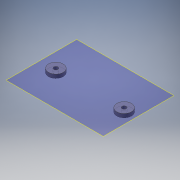
# Autodesk Inventor part: ChassisPrototypeA3
Saved by Autodesk Inventor 2017 (Build 210142000, 142)
## iProperties
Created: 2018-04-24
Part Number: ChassisPrototypeA3
Material: Generic
Document SubType Name: Modeling
Designer: MtgSaber
Mass: 3.50044 g
Surface Area: 26.3822 cm^2
Volume: 3.50044 cm^3
Density: 1 g/cm^3
Appearance: Default
Author: MtgSaber
Autodesk Inventor part; units mm, degrees
ref_plane "YZ Plane" through (0, 0, 0) normal (1, 0, 0) x (0, 1, 0)
ref_plane "Work Plane1" through (-38.4302, 0, 40.64) normal (0, -1, 0) x (-1, 0, 0)
sketch "Sketch1" plane through (-38.4302, 0, 40.64) normal (0, -1, 0) x (-1, 0, 0)
  circle A0 centre (29.6799, 0) radius 1.8288 construction
  circle A1 centre (-29.6799, 0) radius 1.8288 construction
  line L0 (-34.4805, -7.5946) -> (34.4805, -7.5946) construction
  line L1 (34.4805, -7.5946) -> (34.4805, -19.2786) construction
  line L2 (34.4805, -19.2786) -> (-34.4805, -19.2786) construction
  line L3 (-34.4805, -19.2786) -> (-34.4805, -7.5946) construction
  line L4 (34.4805, 7.5946) -> (-34.4805, 7.5946) construction
  line L5 (-34.4805, 7.5946) -> (-34.4805, 19.2786) construction
  line L6 (-34.4805, 19.2786) -> (34.4805, 19.2786) construction
  line L7 (34.4805, 19.2786) -> (34.4805, 7.5946) construction
  line L8 (-38.4302, 27.94) -> (38.4302, 27.94) construction
  line L9 (-38.4302, -27.94) -> (-38.4302, 27.94) construction
  line L10 (38.4302, -27.94) -> (-38.4302, -27.94) construction
  line L11 (38.4302, 27.94) -> (38.4302, -27.94) construction
  circle A2 centre (-29.6799, 0) radius 1.8288
  circle A3 centre (29.6799, 0) radius 1.8288
  circle A4 centre (29.6799, 0) radius 6.35
  circle A5 centre (-29.6799, 0) radius 6.35
  point P0 (-38.4302, 40.64)
  dimension "d0" = 12.7
  dimension "d1" = 12.7
  constraints: 4 centre point, 4 coincident, 2 concentric
  measures "d0" diameter of A4
  measures "d1" diameter of A5
extrude "Extrusion1" add sketch "Sketch1" along normal blind 3.175
ref_plane "Work Plane2" through (-76.8604, 0, 40.64) normal (0, 0, 1) x (1, 0, 0)
sketch "Sketch2" plane through (-76.8604, 0, 40.64) normal (0, 0, 1) x (1, 0, 0)
  line L0 (10.5791, -3.175) -> (6.9215, -3.175) construction
  line L1 (6.9215, 0) -> (10.5791, 0) construction
  line L2 (69.9389, -3.175) -> (66.2813, -3.175) construction
  line L3 (66.2813, 0) -> (69.9389, 0) construction
  line L4 (6.9215, 0) -> (10.5791, 0) construction
  line L5 (8.7503, 0) -> (68.1101, 0) construction
  line L6 (-4.3871, -3.175) -> (85.3512, -3.175) construction
  circle A0 centre (38.4302, -9.525) radius 2.0574
  circle A1 centre (38.4302, -9.525) radius 6.35 construction
  line L7 (38.4302, 0) -> (38.4302, -31.2723) construction
  circle A2 centre (51.1302, -9.525) radius 2.0574
  arc A3 (51.1302, -15.875) -> (57.4802, -9.525) centre (51.1302, -9.525) ccw
  circle A4 centre (25.7302, -9.525) radius 2.0574
  arc A5 (19.3802, -9.525) -> (25.7302, -15.875) centre (25.7302, -9.525) ccw
  line L8 (25.7302, -15.875) -> (51.1302, -15.875)
  line L9 (19.3802, -3.175) -> (57.4802, -3.175)
  line L10 (19.3802, -9.525) -> (19.3802, -3.175)
  line L11 (57.4802, -9.525) -> (57.4802, -3.175)
  point P0 (76.8604, 0)
  point P1 (25.7302, -3.175)
  point P2 (51.1302, -3.175)
  dimension "d4" = 3.175
  dimension "d5" = 4.1148
  dimension "d6" = 12.7
  dimension "d7" = 4.1148
  dimension "d8" = 12.7
  constraints: 14 end point, 7 point on line, 6 centre point, 6 tangent, 4 point on circle, 3 coincident, 3 midpoint, 2 horizontal, 2 perpendicular, 2 symmetric about line, 1 parallel, 1 vertical, 2 other
  measures "d4" distance between parallel lines of L5 L6
  measures "d5" diameter of A0
  measures "d6" diameter of A1
  measures "d7" diameter of A2
  measures "d8" diameter of A3
extrude "Extrusion2" add sketch "Sketch2" along normal mid plane 4.7625
sketch "Sketch3" plane through (-68.1101, 0, 40.64) normal (0, 1, 0) x (1, 0, 0)
  circle A0 centre (0, 0) radius 6.35 construction
  circle A1 centre (59.3598, 0) radius 6.35 construction
  line L0 (10.6299, 2.3813) -> (48.7299, 2.3813) construction
  line L1 (48.7299, -2.3812) -> (10.6299, -2.3812) construction
  line L2 (5.8866, 2.3813) -> (53.4732, 2.3813)
  line L3 (5.8866, -2.3812) -> (53.4732, -2.3812)
  circle A2 centre (0, 0) radius 1.8288 construction
  arc A3 (5.8866, -2.3812) -> (5.8866, 2.3813) centre (0, 0) ccw
  circle A4 centre (59.3598, 0) radius 1.8288 construction
  arc A5 (53.4732, 2.3813) -> (53.4732, -2.3812) centre (59.3598, 0) ccw
  point P0 (68.1101, 40.64)
  constraints: 8 point on circle, 4 end point, 2 centre point, 2 coincident, 2 collinear
extrude "Extrusion3" add sketch "Sketch3" against normal up to surface (3.175 mm away)
fillet "Fillet1" radius 3.175 2 edges at (-19.3802, -3.175, 40.64) (-57.4802, -3.175, 40.64)
body "Solid1"
